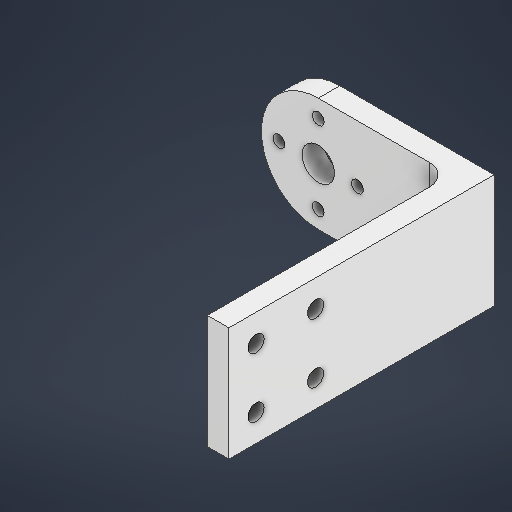
# Autodesk Inventor part: L2
Saved by Autodesk Inventor 2026.1 (Build 301233000, 233)
## iProperties
Created: 2025-09-17
Part Number: L2
Material: Generic
Document SubType Name: Modeling
Designer: emanuel
Density: 1 g/cm^3
Appearance: Default
Author: emanuel
Autodesk Inventor part; units mm, degrees
ref_plane "YZ Plane" through (0, 0, 0) normal (1, 0, 0) x (0, 1, 0)
ref_plane "XZ Plane" through (0, 0, 0) normal (0, 1, 0) x (-1, 0, 0)
ref_plane "XY Plane" through (0, 0, 0) normal (0, 0, 1) x (1, 0, 0)
sketch "Sketch1" plane through (0, 0, 0) normal (0, 1, 0) x (-1, 0, 0)
  line L0 (0, 0) -> (0, -45)
  line L1 (0, -45) -> (35, -45)
  line L2 (35, -45) -> (35, -49)
  line L3 (35, -49) -> (-4, -49)
  line L4 (-4, -49) -> (-4, 0)
  line L5 (-4, 0) -> (0, 0)
  dimension "d0" = 45
  dimension "d1" = 35
  dimension "d2" = 4
  dimension "d3" = 39
  constraints: 12 end point, 4 perpendicular, 1 parallel, 1 vertical
  measures "d0" distance of L0.start L0.end
  measures "d1" distance of L0.end L1.end
  measures "d2" distance of L1.end L2.end
  measures "d3" distance of L2.end L3.end
extrude "Extrusion1" add sketch "Sketch1" along normal blind 21
sketch "Sketch2" plane through (4, 0, 0) normal (1, 0, 0) x (0, 0, -1)
  line L0 (0, 21) -> (49, 21) projected
  line L1 (0, 21) -> (5, 21)
  line L2 (5, 21) -> (5, 16)
  line L3 (5, 16) -> (0, 16)
  line L4 (0, 16) -> (0, 21)
  line L5 (5, 16) -> (16, 16)
  line L6 (16, 16) -> (16, 5)
  line L7 (16, 5) -> (5, 5)
  line L8 (5, 5) -> (5, 16)
  circle A0 centre (5, 16) radius 1.5
  circle A1 centre (16, 16) radius 1.5
  circle A2 centre (5, 5) radius 1.5
  circle A3 centre (16, 5) radius 1.5
  point P0 (0, 0)
  dimension "d6" = 5
  dimension "d7" = 5
  dimension "d8" = 11
  dimension "d9" = 11
  dimension "d10" = 3
  dimension "d11" = 3
  dimension "d12" = 3
  dimension "d13" = 3
  constraints: 16 end point, 4 centre point, 4 coincident, 4 parallel, 2 horizontal, 2 perpendicular
  measures "d6" distance of L2.end L3.end
  measures "d7" distance of L1.end L2.end
  measures "d8" distance of L6.end L7.end
  measures "d9" distance of L5.end L6.end
  measures "d10" diameter of A0
  measures "d11" diameter of A1
  measures "d12" diameter of A2
  measures "d13" diameter of A3
extrude "Extrusion2" cut sketch "Sketch2" against normal blind 21 contours A0 L5 L2 | L2 L3 A0 | L3 L8 A0 | L5 A0 L8 | A1 L6 L5 | L5 L6 A1 | A2 L7 L8 | L8 L7 A2 | A3 L7 L6 | L6 L7 A3
sketch "Sketch3" plane through (-35, 0, -45) normal (0, 0, 1) x (1, 0, 0)
  line L0 (0, 0) -> (0, 21) projected
  line L1 (0, 10.5) -> (10.5, 10.5)
  circle A0 centre (10.5, 10.5) radius 10.5
  line L2 (0, 21) -> (10.5, 21)
  line L3 (10.5, 21) -> (10.5, 0)
  line L4 (10.5, 0) -> (0, 0)
  line L5 (0, 0) -> (0, 21)
  circle A1 centre (10.5, 10.5) radius 8
  circle A2 centre (10.5, 10.5) radius 6.5
  line L6 (10.5, 18.5) -> (10.5, 17)
  line L7 (10.5, 4) -> (10.5, 2.5)
  line L8 (2.5, 10.5) -> (4, 10.5)
  line L9 (10.5, 10.5) -> (18.5, 10.5)
  line L10 (18.5, 10.5) -> (17, 10.5)
  circle A3 centre (10.5, 17.75) radius 1.1
  circle A4 centre (3.25, 10.5) radius 1.1
  circle A5 centre (17.75, 10.5) radius 1.1
  circle A6 centre (10.5, 3.25) radius 1.1
  circle A7 centre (10.5, 10.5) radius 3
  point P0 (35, 0)
  point P1 (10.5, 21)
  dimension "d16" = 10.5
  dimension "d17" = 16
  dimension "d18" = 13
  dimension "d19" = 2.2
  dimension "d20" = 2.2
  dimension "d21" = 2.2
  dimension "d22" = 2.2
  dimension "d23" = 6
  constraints: 20 end point, 10 point on circle, 8 centre point, 8 point on line, 5 midpoint, 4 coincident, 2 horizontal, 2 parallel, 1 perpendicular
  measures "d16" distance of L1.start L1.end
  measures "d17" diameter of A1
  measures "d18" diameter of A2
  measures "d19" diameter of A3
  measures "d20" diameter of A4
  measures "d21" diameter of A5
  measures "d22" diameter of A6
  measures "d23" diameter of A7
extrude "Extrusion3" cut sketch "Sketch3" against normal blind 21 contours L0 A0 L4 | L0 L2 A0 | A4 A1 L1 | L1 A1 A4 | A6 A1 L3 | L3 A1 A6 | A1 A4 A2 L1 | L1 A2 A4 A1 | A3 A1 L3 | L3 A1 A3 | A1 A6 A2 L3 | L3 A2 A6 A1 | A2 A4 L1 | L1 A4 A2 | A1 L3 A2 A3 | A1 A3 A2 L3 | A2 A6 L3 | L3 A6 A2 | A5 A2 L9 A1 | A1 A5 | A2 L3 A3 | A2 A3 L3 | A1 L9 A2 A5 | A5 L9 A2 | A7 L3 L1 | L1 L3 A7 | A2 L9 A5 | L3 L9 A7 | L3 A7 L9
fillet "Fillet1" radius 4 1 edges at (0, 10.5, -45)
body "Solid1"
